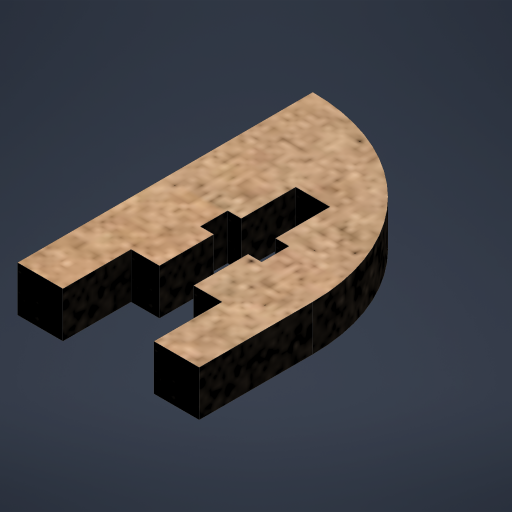
# Autodesk Inventor part: Lever
Saved by Autodesk Inventor 2024.1 (Build 281209000, 209)
## iProperties
Created: 2023-05-21
Part Number: Lever
Material: MDF Medium Density Fiberboard
Document SubType Name: Modeling
Designer: jaege
Density: 0.8 g/cm^3
Appearance: Cardboard - Chipboard 1
Author: jaege
Autodesk Inventor part; units mm, degrees
ref_plane "YZ Plane" through (0, 0, 0) normal (1, 0, 0) x (0, 1, 0)
ref_plane "XZ Plane" through (0, 0, 0) normal (0, 1, 0) x (-1, 0, 0)
ref_plane "XY Plane" through (0, 0, 0) normal (0, 0, 1) x (1, 0, 0)
sketch "Sketch1" plane through (0, 0, 0) normal (0, 1, 0) x (-1, 0, 0)
  line L0 (8, 13) -> (8, 7)
  line L1 (8, 7) -> (8, 7)
  line L2 (8, 7) -> (8, -13)
  line L3 (8, -13) -> (-8, -13)
  line L4 (-8, -13) -> (-8, 13)
  line L5 (-8, 13) -> (-4, 13)
  line L6 (-4, 13) -> (-4, 7)
  line L7 (-4, 7) -> (4, 7)
  line L8 (4, 7) -> (4, 13)
  line L9 (4, 13) -> (8, 13)
  line L10 (8, -13) -> (-8, 13) construction
  line L11 (1.5, 7) -> (-1.5, 7)
  line L12 (-1.5, 7) -> (-1.5, -5)
  line L13 (-1.5, -5) -> (1.5, -5)
  line L14 (1.5, -5) -> (1.5, 7)
  line L15 (2.7, -0.2) -> (-2.7, -0.2)
  line L16 (-2.7, -0.2) -> (-2.7, 2.2)
  line L17 (-2.7, 2.2) -> (2.7, 2.2)
  line L18 (2.7, 2.2) -> (2.7, -0.2)
  point P0 (0, 0)
  point P1 (0, 0)
  point P2 (0, 2.2)
  point P3 (0, -5)
  point P4 (-2.7, 1)
  point P5 (-1.5, 1)
  point P6 (0, 7)
  point P7 (1.5, 2.2)
  point P8 (1.5, -0.2)
  point P9 (-1.5, -0.2)
  point P10 (-1.5, 2.2)
  dimension "d0" = 6
  dimension "d1" = 4
  dimension "d3" = 0
  dimension "d4" = 4
  dimension "d5" = 20
  dimension "d10" = 8
  dimension "d11" = 3
  dimension "d12" = 12
  dimension "d13" = 5.4
  dimension "d14" = 2.4
  constraints: 38 end point, 9 perpendicular, 6 midpoint, 4 parallel, 3 horizontal, 2 horizontal alignment, 2 point on line, 2 vertical, 2 vertical alignment, 1 coincident
  measures "d0" distance of L0.start L0.end
  measures "d1" distance of L8.end L0.start
  measures "d3" distance of L0.end L1.end
  measures "d4" distance of L4.end L5.end
  measures "d5" distance between parallel lines of L3 L1
  measures "d10" distance between parallel lines of L8 L6
  measures "d11" distance of L13.end L12.end
  measures "d12" distance of L12.end L11.end
  measures "d13" distance of L16.end L17.end
  measures "d14" distance of L15.end L16.end
extrude "Extrusion1" add sketch "Sketch1" along normal blind 4 contours L0 L2 L3 L4 L5 L6 L7 L12 L17 L16 L15 L13 L14 L18 L8 L9
fillet "Fillet1" radius 16 1 edges at (8, 2, -13)
body "Solid1"
